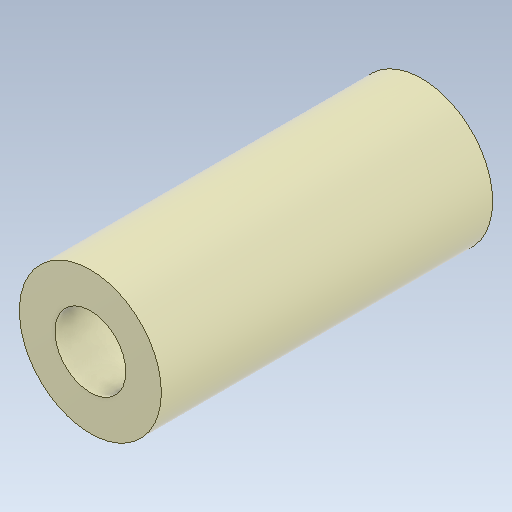
# Autodesk Inventor part: PEAKスペーサーm3-14 丸形両雌ねじ
Saved by Autodesk Inventor 2020.2 (Build 242310000, 310)
## iProperties
Created: 2020-05-15
Part Number: PEAKスペーサーm3-14 丸形両雌ねじ
Material: PAEK 樹脂
Document SubType Name: Modeling
Designer: mozar
Mass: 0.391882 g
Surface Area: 4.38252 cm^2
Volume: 0.296881 cm^3
Density: 1.32 g/cm^3
Appearance: 滑らか - 灰色
Author: mozar
Autodesk Inventor part; units mm, degrees
ref_plane "YZ Plane" through (0, 0, 0) normal (1, 0, 0) x (0, 1, 0)
ref_plane "XZ Plane" through (0, 0, 0) normal (0, 1, 0) x (-1, 0, 0)
ref_plane "XY Plane" through (0, 0, 0) normal (0, 0, 1) x (1, 0, 0)
sketch "スケッチ1" plane through (0, 0, 0) normal (0, 0, 1) x (1, 0, 0)
  circle A0 centre (0, 0) radius 3
  circle A1 centre (0, 0) radius 1.5
  dimension "d0" = 6
  dimension "d1" = 3
  constraints: 2 centre point, 2 coincident
  measures "d0" diameter of A0
  measures "d1" diameter of A1
extrude "押し出し1" add sketch "スケッチ1" against normal blind 14
